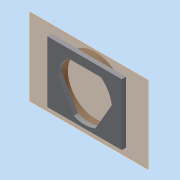
# Autodesk Inventor part: 20_Cube_Insert_Z-Focus_objectivemount
Saved by Autodesk Inventor 2019.4 (Build 234330000, 330)
## iProperties
Created: 2020-12-08
Part Number: 20_Cube_Insert_Z-Focus_objectivemount
Material: Generic
Document SubType Name: Modeling
Designer: diederichbenedict
Density: 1 g/cm^3
Appearance: Default
Author: diederichbenedict
Autodesk Inventor part; units mm, degrees
ref_plane "YZ Plane" through (0, 0, 0) normal (1, 0, 0) x (0, 1, 0)
ref_plane "XZ Plane" through (0, 0, 0) normal (0, 1, 0) x (-1, 0, 0)
ref_plane "XY Plane" through (0, 0, 0) normal (0, 0, 1) x (1, 0, 0)
ref_plane "Work Plane1" through (0, 0, 0) normal (0, 0, 1) x (1, 0, 0)
sketch "Sketch1" plane through (0, 0, 0) normal (0, 0, 1) x (1, 0, 0)
  circle A0 centre (11.8906, 0.2887) radius 14 construction
  line L0 (-4.1094, 7.6362) -> (-12.7094, 0.2473) construction
  line L1 (-5.7094, 0.2473) -> (-12.7094, 0.2473) construction
  line L2 (-5.7094, -6.0861) -> (-5.7094, 0.2473) construction
  line L3 (-6.0301, -6.0861) -> (-5.7094, -6.0861) construction
  line L4 (-6.0301, -6.0861) -> (-4.1094, -7.5697) construction
  line L5 (-4.1094, -7.5697) -> (-4.1094, -15.7113) construction
  line L6 (-4.1094, -15.7113) -> (27.8906, -15.7113) construction
  line L7 (27.8906, -15.7113) -> (27.8906, -7.5697) construction
  line L8 (29.8113, -6.0861) -> (27.8906, -7.5697) construction
  line L9 (29.4906, -6.0861) -> (29.8113, -6.0861) construction
  line L10 (29.4906, 0.2473) -> (29.4906, -6.0861) construction
  line L11 (36.4906, 0.2473) -> (29.4906, 0.2473) construction
  line L12 (27.8906, 7.6362) -> (36.4906, 0.2473) construction
  line L13 (27.8906, 7.6362) -> (27.8906, 16.2887) construction
  line L14 (27.8906, 16.2887) -> (-4.1094, 16.2887) construction
  line L15 (-4.1094, 16.2887) -> (-4.1094, 7.6362) construction
  circle A1 centre (11.8906, 0.2887) radius 13.9
  circle A2 centre (11.8906, 0.2887) radius 12.5
  point P0 (0, 0)
  dimension "d0" = 27.8
  dimension "d1" = 25
  constraints: 2 centre point, 2 coincident
  measures "d0" diameter of A1
  measures "d1" diameter of A2
extrude "Extrusion1" add sketch "Sketch1" against normal blind 3 draft -2
sketch "Sketch2" plane through (11.8906, 0.2887, 0) normal (0, 0, 1) x (1, 0, 0)
  circle A0 centre (0, 0) radius 13.9 projected
  circle A1 centre (0, 0) radius 12.5 projected
  line L0 (17, -14) -> (-17, -14)
  line L1 (-17, -14) -> (-17, 14)
  line L2 (-17, 14) -> (17, 14)
  line L3 (17, 14) -> (17, -14)
  line L4 (17, -14) -> (-17, 14) construction
  line L5 (-17, -14) -> (17, 14) construction
  circle A2 centre (0, 0) radius 10.05 construction
  line L6 (-7.4329, 10.05) -> (7.4329, 10.05)
  line L7 (-12.42, 1.4121) -> (-4.9871, -11.4621)
  line L8 (4.9871, -11.4621) -> (12.42, 1.4121)
  point P0 (-11.8906, -0.2887)
  dimension "d4" = 34
  dimension "d5" = 28
  dimension "d8" = 20.1
  dimension "d9" = 60
  dimension "d10" = 60
  dimension "d11" = 0
  constraints: 18 end point, 6 point on circle, 3 midpoint, 3 tangent, 2 horizontal, 2 parallel, 1 centre point, 1 perpendicular
  measures "d4" distance of L1.end L2.end
  measures "d5" distance of L0.end L1.end
  measures "d8" diameter of A2
  measures "d9" angle of L7 L6
  measures "d10" angle of L6 L8
  measures "d11" distance of A0.centre A2.centre
extrude "Extrusion2" add sketch "Sketch2" along normal blind 2 contours A0 | A1 L8 | L6 A1 | A1 L7 | L0 L1 L2 L3
body "Solid1"
